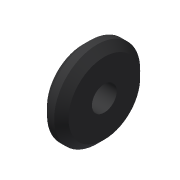
# Autodesk Inventor part: Thumb Screw
Saved by Autodesk Inventor 2022 Beta2 (Build 260130000, 130) ContinuousBuild 0
## iProperties
Created: 2006-01-31
Part Number: Thumb Screw
Document SubType Name: Modeling
Designer: landrews
Stock Number: Thumb Screw
Density: 1 g/cm^3
Material: Generic
Appearance: Generic
Author: landrews
Autodesk Inventor part; units mm, degrees
ref_plane "YZ Plane" through (0, 0, 0) normal (1, 0, 0) x (0, 1, 0)
ref_plane "XZ Plane" through (0, 0, 0) normal (0, 1, 0) x (-1, 0, 0)
ref_plane "XY Plane" through (0, 0, 0) normal (0, 0, 1) x (1, 0, 0)
sketch "Sketch1" plane through (0, 0, 0) normal (0, 1, 0) x (-1, 0, 0)
  line L0 (-12.6754, 0) -> (9.1433, 0) projected
  line L1 (0, -1.2) -> (0, 15.6) projected
  line L2 (0, 0) -> (0, 6.5)
  arc A0 (-2, 8.5) -> (0, 6.5) centre (0, 8.5) ccw
  line L3 (-2, 8.5) -> (-2, 10)
  line L4 (-2, 10) -> (-4, 12)
  line L5 (-4, 12) -> (-6, 12)
  line L6 (-6, 12) -> (-8, 10)
  line L7 (-8, 10) -> (-8, 0)
  line L8 (-8, 0) -> (0, 0)
  line L9 (0, 6.5) -> (7.5848, 6.5) construction
  dimension "d0" = 90
  dimension "d1" = 6.5
  dimension "d2" = 2
  dimension "d3" = 2
  dimension "d4" = 2
  dimension "d5" = 6
  dimension "d6" = 12
  dimension "d7" = 2
  dimension "d8" = 135
  constraints: 16 end point, 4 point on line, 2 parallel, 2 perpendicular, 2 point on circle, 2 tangent, 1 centre point, 1 collinear
  measures "d0" angle of L6 L4
  measures "d1" distance of L2.start L2.end
  measures "d2" radius of A0
  measures "d3" distance between parallel lines of L1 L3
  measures "d4" horizontal distance of L5.end L6.end
  measures "d5" distance between parallel lines of L7 L3
  measures "d6" distance between parallel lines of L0 L5
  measures "d7" horizontal distance of L3.end L4.end
  measures "d8" angle of L7 L6
revolve "Revolution1" add sketch "Sketch1" angle 360 about axis through (8, 0, 0) along (-1, 0, 0)
hole "Hole1" at (0, 0, 0) direction (1, 0, 0) diameter 6.917 end through all
body "Solid1"
